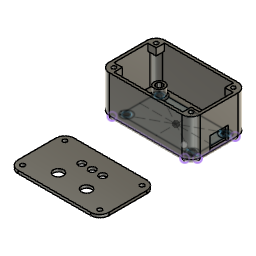
Sound Unit - No Holes (Autodesk Fusion 360 design; units mm, degrees)
Autodesk Fusion 360 part; units mm, degrees
note: some values were not read from the file. Set by a fixed rule: which face or edge a step refers to.
sketch "Sketch1" plane through (0, 0, 0) normal (0, 0, 1) x (1, 0, 0)
  line L0 (6.5, 0) -> (58.5, 0)
  line L1 (65, -6.5) -> (65, -33.5)
  line L2 (58.5, -40) -> (6.5, -40)
  line L3 (0, -33.5) -> (0, -6.5)
  arc A0 (0, -33.5) -> (6.5, -40) centre (6.5, -33.5) ccw
  arc A1 (6.5, 0) -> (0, -6.5) centre (6.5, -6.5) ccw
  arc A2 (65, -6.5) -> (58.5, 0) centre (58.5, -6.5) ccw
  arc A3 (58.5, -40) -> (65, -33.5) centre (58.5, -33.5) ccw
  point P0 (65, 0)
  point P1 (6.5, -33.5)
  point P2 (30.568, -50.8814)
  dimension "d1" = 65
  dimension "d2" = 40
  dimension "d294" = 6.5
  constraint horizontal L0
  constraint vertical L1
  constraint horizontal L2
  constraint vertical L3
  constraint tangent L2 A0
  constraint tangent L3 A0
  constraint coincident origin L0
  constraint coincident origin L3
  constraint tangent L0 A1
  constraint tangent L3 A1
  constraint equal A0 A1
  constraint coincident P0 L0
  constraint coincident P0 L1
  constraint tangent L0 A2
  constraint tangent L1 A2
  constraint equal A0 A2
  constraint tangent L1 A3
  constraint tangent L2 A3
  constraint equal A0 A3
  constraint coincident P1 A0.centre
  measures "d1" distance of origin P0
  measures "d2" distance of L0 L2
  measures "d294" radius of A0
extrude "Extrude1" add sketch "Sketch1" along normal blind 30 makes body 1
sketch "Sketch2" plane through (0, 0, 0) normal (-1, 0, 0) x (0, -1, 0)
shell "Shell1" thickness 2 removed faces 1 at (41.1667, -26.6667, 30) on bodies 1
sketch "Sketch3" plane through (0, 0, 2) normal (0, 0, 1) x (-1, 0, 0)
  circle A0 centre (-10.6, 31.7) radius 2.3971
  line L0 (-60, 6) -> (-60, 34)
  line L1 (-8.3, 34) -> (-8.3, 6)
  circle A1 centre (-57.7, 8.3) radius 3.8971
  circle A2 centre (-10.6, 31.7) radius 3.8971
  line L2 (-60, 34) -> (-8.3, 6) construction
  line L3 (-8.3, 34) -> (-60, 6) construction
  circle A3 centre (-10.6, 8.3) radius 2.3971
  line L4 (-34.15, 6) -> (-34.15, 34) construction
  line L5 (-8.3, 6) -> (-60, 6)
  line L6 (-60, 34) -> (-8.3, 34)
  circle A4 centre (-10.6, 8.3) radius 3.8971
  circle A5 centre (-57.7, 8.3) radius 2.3971
  line L7 (-8.3, 20) -> (-60, 20) construction
  circle A6 centre (-57.7, 31.7) radius 3.8971
  circle A7 centre (-57.7, 31.7) radius 2.3971
  line L8 (-53.8029, 31.6996) -> (-61.5971, 31.6996)
  line L9 (-53.8029, 8.3) -> (-61.5971, 8.3)
  line L10 (-58.5, 38) -> (-6.5, 38)
  line L11 (-63, 6.5) -> (-63, 33.5)
  point P0 (-34.15, 20)
  point P1 (-49.8386, 29.9282)
  dimension "d21" = 51.7
  dimension "d22" = 28
  dimension "d23" = 2.3
  dimension "d24" = 2.3
  dimension "d27" = 1.5
  dimension "d349" = 4
  dimension "d350" = 3
  constraint horizontal L6
  constraint perpendicular L1 L6
  constraint parallel L5 L6
  constraint parallel L0 L1
  constraint coincident P0 L2
  constraint coincident P0 L3
  constraint midpoint L4.start L5
  constraint midpoint L4.end L6
  constraint midpoint L7.start L1
  constraint midpoint L7.end L0
  constraint symmetric A0 A3 L7
  constraint symmetric A3 L4 A5
  constraint symmetric A0 L4 A7
  constraint concentric A3 A4
  constraint symmetric A2 A4 L7
  constraint symmetric A1 L4 A4
  constraint symmetric A2 L4 A6
  constraint coincident A6 L8.start
  constraint coincident A6 L8.end
  constraint perpendicular L0 L8
  constraint coincident A1 L9.start
  constraint coincident A1 L9.end
  constraint horizontal L9
  measures "d21" distance of L1.end L0.start
  measures "d22" distance of L0.start L0.end
  measures "d23" distance of A3.centre L5
  measures "d24" distance of A3.centre L1
  measures "d27" distance of A3 A4
  measures "d349" distance of L6 L10
  measures "d350" distance of L0 L11
extrude "Extrude4" cut sketch "Sketch3" against normal up to surface (2 mm away) contours A0 L1 | A0 L1 L6 | A0 L6 | L1 A3 | L1 A3 L5 | L0 L6 A7 L8 | L6 A7 | A3 L5 | L0 A7 L8 | L0 A7 L8 | L0 A7 L8 | L5 A5 | L0 L5 A5 L9 | L0 A5 L9 | L0 A5 L9 | L0 A5 L9 picked at (-11.2582, 32.2325) picked at (-11.0806, 8.835) bodies 1
extrude "Extrude3" cut sketch "Sketch3" against normal up to surface (1.5 mm away) from surface at -0.5 contours A0 L1 | A0 L1 A2 L6 | A0 L1 L6 | A0 L1 L6 | A0 L1 A2 L6 | A0 L6 | L1 A3 L5 A4 | L1 A3 L5 A4 | L6 A6 A7 L8 | L0 L6 A6 A7 L8 | L1 A3 | L1 A3 L5 | L0 L6 A7 L8 | L6 A7 | L0 A6 A7 L8 | L0 A6 A7 L8 | L1 A3 L5 | A3 L5 | A1 L5 A5 L9 | L0 A1 L5 A5 L9 | L0 L6 A7 | L0 A7 L8 | L0 A7 L8 | L0 A7 L8 | L0 A1 A5 L9 | L0 A1 A5 L9 | L5 A5 | L0 L5 A5 L9 | L0 A5 L9 | L0 A5 L9 | L0 A5 L9 | L0 L5 A5 bodies 1
extrude "Extrude5" add sketch "Sketch3" along normal blind 6.5 contours A0 L1 | A0 L1 A2 L6 | A0 L1 L6 | A0 L1 A2 L6 | A0 L6 | L1 A3 L5 A4 | L1 A3 L5 A4 | L6 A6 A7 L8 | L0 L6 A6 A7 L8 | L1 A3 | L6 A7 | L1 A3 L5 | A3 L5 | A1 L5 A5 L9 | L0 A1 L5 A5 L9 | L0 L6 A7 | L0 A7 L8 | L5 A5 | L0 A5 L9 | L0 L5 A5 picked at (-8.7062, 33.5938) picked at (-8.7062, 6.4062) picked at (-60.0611, 31.7756) picked at (-60.0611, 8.2241) bodies 1
chamfer "Chamfer1" distance 1 angle 45 4 edges at (14.2334, -9.7092, 2) (14.2334, -33.1092, 2) (57.7, -35.5971, 2) (57.7, -4.4029, 2) on bodies 1
sketch "Sketch5" plane through (63, 0, 0) normal (-1, 0, 0) x (0, -1, 0)
  line L0 (33.5, 30) -> (6.5, 30)
  line L1 (13.5, 13.5, -2) -> (26.5, 13.5, -2)
  line L2 (26.5, 13.5, -2) -> (26.5, 3.5, -2)
  line L3 (26.5, 3.5, -2) -> (13.5, 3.5, -2)
  line L4 (13.5, 3.5, -2) -> (13.5, 13.5, -2)
  line L5 (26.5, 13.5, -2) -> (13.5, 3.5, -2) construction
  line L6 (26.5, 3.5, -2) -> (13.5, 13.5, -2) construction
  line L7 (33.5, 0) -> (33.5, 30)
  line L8 (33.5, 30, -2) -> (6.5, 0, -2) construction
  line L9 (6.5, 0, -2) -> (6.5, 30, -2) construction
  line L10 (6.5, 30, -2) -> (33.5, 0, -2) construction
  line L11 (6.5, 2) -> (33.5, 2)
  line L12 (6.5, 0, -2) -> (33.5, 0, -2)
  point P0 (20, 12.5)
  point P1 (33.5, 30)
  point P2 (6.5, 0)
  point P3 (6.5, 30)
  point P4 (33.5, 0)
  point P5 (20, 12.5)
  dimension "d46" = 13
  dimension "d47" = 10
  dimension "d356" = 3.5
  constraint coincident P1 L0.start
  constraint coincident P3 L0.end
  constraint coincident P4 L7.start
  constraint coincident P5 P0
extrude "Extrude13" cut sketch "Sketch5" along normal up to surface (2 mm away) contours L1 L2 L3 L4 in plane through (65, 0, 0) normal (-1, 0, 0) bodies 1
sketch "Sketch6" plane through (0, -40, 0) normal (0, -1, 0) x (1, 0, 0)
  line L0 (58.5, 30) -> (6.5, 30)
  line L1 (60, 2) -> (8.3, 2)
  line L2 (6.5, 0) -> (58.5, 0)
  line L3 (58.5, 0) -> (58.5, 30)
  line L4 (6.5, 30) -> (6.5, 0)
sketch "Sketch7" plane through (0, 0, 30) normal (0, 0, 1) x (-1, 0, 0)
  arc A0 (-6.5, 0) -> (0, 6.5) centre (-6.5, 6.5) ccw construction
  circle A1 centre (-4.9038, 4.9038) radius 1.5
  arc A2 (-6.5, 2) -> (-2, 6.5) centre (-6.5, 6.5) ccw
  line L0 (-1.9038, 1.9038) -> (-7.9038, 1.9038) construction
  line L1 (-7.9038, 1.9038) -> (-7.9038, 7.9038) construction
  line L2 (-7.9038, 7.9038) -> (-1.9038, 7.9038) construction
  line L3 (-1.9038, 7.9038) -> (-1.9038, 1.9038) construction
  line L4 (-1.9038, 1.9038) -> (-7.9038, 7.9038) construction
  line L5 (-1.9038, 7.9038) -> (-7.9038, 1.9038) construction
  line L6 (-7.9038, 7.9038) -> (-2, 7.9038)
  line L7 (-7.9038, 2) -> (-7.9038, 7.9038)
  line L8 (-7.9038, 2) -> (-6.5, 2)
  line L9 (-2, 7.9038) -> (-2, 6.5)
  line L10 (-63.0962, 1.9038) -> (-57.0962, 1.9038) construction
  line L11 (-57.0962, 1.9038) -> (-57.0962, 7.9038) construction
  line L12 (-57.0962, 7.9038) -> (-63.0962, 7.9038) construction
  line L13 (-63.0962, 7.9038) -> (-63.0962, 1.9038) construction
  arc A3 (-65, 6.5) -> (-58.5, 0) centre (-58.5, 6.5) ccw construction
  line L14 (-57.0962, 7.9038) -> (-63.0962, 1.9038) construction
  line L15 (-57.0962, 1.9038) -> (-63.0962, 7.9038) construction
  circle A4 centre (-60.0962, 4.9038) radius 1.5
  line L16 (-57.0962, 2) -> (-57.0962, 7.9038)
  line L17 (-63, 7.9038) -> (-57.0962, 7.9038)
  line L18 (-63, 7.9038) -> (-63, 6.5)
  line L19 (-57.0962, 2) -> (-58.5, 2)
  arc A5 (-63, 6.5) -> (-58.5, 2) centre (-58.5, 6.5) ccw
  line L20 (-63.0962, 38.0962) -> (-57.0962, 38.0962) construction
  line L21 (-57.0962, 38.0962) -> (-57.0962, 32.0962) construction
  line L22 (-57.0962, 32.0962) -> (-63.0962, 32.0962) construction
  line L23 (-63.0962, 32.0962) -> (-63.0962, 38.0962) construction
  arc A6 (-58.5, 40) -> (-65, 33.5) centre (-58.5, 33.5) ccw construction
  line L24 (-63.0962, 32.0962) -> (-57.0962, 38.0962) construction
  line L25 (-57.0962, 32.0962) -> (-63.0962, 38.0962) construction
  circle A7 centre (-60.0962, 35.0962) radius 1.5
  line L26 (-57.0962, 32.0962) -> (-63.0227, 32.0962)
  line L27 (-63.0227, 32.0962) -> (-63, 33.5)
  line L28 (-57.0962, 32.0962) -> (-57.0962, 38.007)
  line L29 (-57.0962, 38.007) -> (-58.5, 38)
  arc A8 (-58.5, 38) -> (-63, 33.5) centre (-58.5, 33.5) ccw
  line L30 (-1.9038, 38.0962) -> (-7.9038, 38.0962) construction
  line L31 (-7.9038, 38.0962) -> (-7.9038, 32.0962) construction
  line L32 (-7.9038, 32.0962) -> (-1.9038, 32.0962) construction
  line L33 (-1.9038, 32.0962) -> (-1.9038, 38.0962) construction
  arc A9 (0, 33.5) -> (-6.5, 40) centre (-6.5, 33.5) ccw construction
  line L34 (-1.9038, 38.0962) -> (-7.9038, 32.0962) construction
  line L35 (-1.9038, 32.0962) -> (-7.9038, 38.0962) construction
  circle A10 centre (-4.9038, 35.0962) radius 1.5
  line L36 (-7.9038, 32.0962) -> (-2, 32.0962)
  line L37 (-2, 32.0962) -> (-2, 33.5)
  line L38 (-7.9038, 32.0962) -> (-7.9038, 38.1423)
  line L39 (-7.9038, 38.1423) -> (-6.5, 38)
  arc A11 (-2, 33.5) -> (-6.5, 38) centre (-6.5, 33.5) ccw
  point P0 (-9.5, -1)
  point P1 (-3.318, 3.318)
  point P2 (-4.9038, 4.9038)
  point P3 (-4.9038, 4.9038)
  point P4 (-3.318, 3.318)
  point P5 (-3.724, 2.9583)
  point P6 (-60.0962, 4.9038)
  point P7 (-58.5, 2)
  point P8 (-63, 6.5)
  point P9 (-61.682, 3.318)
  point P10 (-77.5, 3.8)
  point P11 (-60.0962, 35.0962)
  point P12 (-63, 33.5)
  point P13 (-58.5, 38)
  point P14 (-61.682, 36.682)
  point P15 (-4.9038, 35.0962)
  point P16 (-2, 33.5)
  point P17 (-6.5, 38)
  point P18 (-3.318, 36.682)
  point P19 (-2, 53.1422)
  dimension "d309" = 3
  dimension "d322" = 6
  dimension "d323" = 6
  dimension "d324" = 6
  dimension "d325" = 6
  dimension "d326" = 3
  dimension "d329" = 6
  dimension "d330" = 6
  dimension "d331" = 3
  dimension "d332" = 6
  dimension "d333" = 6
  dimension "d334" = 3
  constraint midpoint P4 A2
  constraint coincident P3 P2
  constraint horizontal L0
  constraint vertical L1
  constraint horizontal L2
  constraint vertical L3
  constraint midpoint A0 L0.start
  constraint midpoint L5 P3
  constraint coincident L2 L6.end
  constraint coincident L1 L7.start
  constraint coincident P4 P1
  constraint coincident A2.start L8.end
  constraint tangent A2 L8
  constraint coincident A2.end L9.end
  constraint tangent A2 L9
  constraint horizontal L10
  constraint vertical L11
  constraint horizontal L12
  constraint vertical L13
  constraint midpoint L10.start A3
  constraint midpoint L15 P6
  constraint coincident P6 A4.centre
  constraint coincident L11 L16.start
  constraint coincident L12 L17.start
  constraint perpendicular L16 L17
  constraint coincident P8 L18.end
  constraint perpendicular L17 L18
  constraint coincident P7 L19.end
  constraint perpendicular L16 L19
  constraint midpoint P9 A5
  constraint horizontal L20
  constraint vertical L21
  constraint horizontal L22
  constraint vertical L23
  constraint midpoint L20.start A6
  constraint midpoint L24 P11
  constraint coincident P11 A7.centre
  constraint coincident L22 L26.end
  constraint coincident P12 L27.end
  constraint coincident L21 L28.end
  constraint coincident P13 L29.end
  constraint midpoint P14 A8
  constraint horizontal L30
  constraint vertical L31
  constraint horizontal L32
  constraint vertical L33
  constraint midpoint L30.start A9
  constraint midpoint L34 P15
  constraint coincident P15 A10.centre
  constraint coincident L32 L36.end
  constraint coincident P16 L37.end
  constraint coincident L31 L38.end
  constraint perpendicular L32 L38
  constraint coincident P17 L39.end
  constraint midpoint P18 A11
  measures "d309" diameter of A1
  measures "d322" distance of L0.start L0.end
  measures "d323" distance of L0.start L2.end
  measures "d324" distance of L10.start L10.end
  measures "d325" distance of L10.start L12.end
  measures "d326" diameter of A4
  measures "d329" distance of L20.start L20.end
  measures "d330" distance of L20.start L22.end
  measures "d331" diameter of A7
  measures "d332" distance of L30.start L30.end
  measures "d333" distance of L30.start L32.end
  measures "d334" diameter of A10
extrude "Extrude8" add sketch "Sketch7" against normal blind 5 bodies 1
sketch "Sketch8" plane through (0, 0, 0) normal (0, 0, 1) x (1, 0, 0)
  line L0 (58.3615, -65.1296) -> (6.3615, -65.1296)
  line L1 (-0.1385, -71.6296) -> (-0.1385, -98.6296)
  line L2 (6.3615, -105.1296) -> (58.3615, -105.1296)
  line L3 (64.8615, -98.6296) -> (64.8615, -71.6296)
  arc A0 (6.3615, -65.1296) -> (-0.1385, -71.6296) centre (6.3615, -71.6296) ccw
  arc A1 (-0.1385, -98.6296) -> (6.3615, -105.1296) centre (6.3615, -98.6296) ccw
  arc A2 (64.8615, -71.6296) -> (58.3615, -65.1296) centre (58.3615, -71.6296) ccw
  arc A3 (58.3615, -105.1296) -> (64.8615, -98.6296) centre (58.3615, -98.6296) ccw
  line L4 (1.7653, -67.0334) -> (62.9576, -103.2258) construction
  line L5 (62.9576, -67.0334) -> (1.7653, -103.2258) construction
  circle A4 centre (4.7653, -70.0334) radius 1.5
  line L6 (1.7653, -67.0334) -> (7.7653, -67.0334) construction
  line L7 (7.7653, -67.0334) -> (7.7653, -73.0334) construction
  line L8 (7.7653, -73.0334) -> (1.7653, -73.0334) construction
  line L9 (1.7653, -73.0334) -> (1.7653, -67.0334) construction
  line L10 (7.7653, -67.0334) -> (1.7653, -73.0334) construction
  line L11 (1.7653, -67.0334) -> (7.7653, -73.0334) construction
  line L12 (62.9576, -67.0334) -> (56.9576, -67.0334) construction
  line L13 (56.9576, -67.0334) -> (56.9576, -73.0334) construction
  line L14 (56.9576, -73.0334) -> (62.9576, -73.0334) construction
  line L15 (62.9576, -73.0334) -> (62.9576, -67.0334) construction
  line L16 (56.9576, -67.0334) -> (62.9576, -73.0334) construction
  line L17 (56.9576, -73.0334) -> (62.9576, -67.0334) construction
  circle A5 centre (59.9576, -70.0334) radius 1.5
  line L18 (62.9576, -103.2258) -> (56.9576, -103.2258) construction
  line L19 (56.9576, -103.2258) -> (56.9576, -97.2258) construction
  line L20 (56.9576, -97.2258) -> (62.9576, -97.2258) construction
  line L21 (62.9576, -97.2258) -> (62.9576, -103.2258) construction
  line L22 (56.9576, -97.2258) -> (62.9576, -103.2258) construction
  line L23 (62.9576, -97.2258) -> (56.9576, -103.2258) construction
  circle A6 centre (59.9576, -100.2258) radius 1.5
  line L24 (1.7653, -103.2258) -> (7.7653, -103.2258) construction
  line L25 (7.7653, -103.2258) -> (7.7653, -97.2258) construction
  line L26 (7.7653, -97.2258) -> (1.7653, -97.2258) construction
  line L27 (1.7653, -97.2258) -> (1.7653, -103.2258) construction
  line L28 (1.7653, -97.2258) -> (7.7653, -103.2258) construction
  line L29 (7.7653, -97.2258) -> (1.7653, -103.2258) construction
  circle A7 centre (4.7653, -100.2258) radius 1.5
  line L30 (20.1684, -78.0671) -> (44.5545, -78.0671) construction
  circle A8 centre (22.2882, -92.1922) radius 3.65
  circle A9 centre (24.8615, -78.0671) radius 2.5
  circle A10 centre (32.3615, -78.0671) radius 2.5
  circle A11 centre (39.8615, -78.0671) radius 2.5
  circle A12 centre (42.4347, -92.1922) radius 3.65
  line L31 (-0.1385, -85.1296) -> (64.8615, -85.1296) construction
  line L32 (32.3615, -65.1296) -> (32.3615, -105.1296) construction
  line L33 (22.2882, -92.1922) -> (42.4347, -92.1922) construction
  line L34 (32.3615, -78.0671) -> (32.3615, -92.1922) construction
  point P0 (4.7653, -70.0334)
  point P1 (59.9576, -70.0334)
  point P2 (59.9576, -100.2258)
  point P3 (4.7653, -100.2258)
  point P4 (32.3615, -85.1296)
  dimension "d179" = 6.5
  dimension "d196" = 40
  dimension "d197" = 65
  dimension "d303" = 3
  dimension "d336" = 6
  dimension "d337" = 6
  dimension "d338" = 6
  dimension "d339" = 6
  dimension "d340" = 3
  dimension "d341" = 6
  dimension "d342" = 6
  dimension "d343" = 3
  dimension "d344" = 6
  dimension "d345" = 6
  dimension "d346" = 3
  dimension "d370" = 5
  dimension "d371" = 5
  dimension "d372" = 5
  dimension "d373" = 7.5
  dimension "d374" = 7.5
  constraint horizontal L0
  constraint vertical L1
  constraint horizontal L2
  constraint vertical L3
  constraint tangent L0 A0
  constraint tangent L1 A0
  constraint tangent L1 A1
  constraint tangent L2 A1
  constraint equal A0 A1
  constraint tangent L0 A2
  constraint tangent L3 A2
  constraint equal A0 A2
  constraint tangent L2 A3
  constraint tangent L3 A3
  constraint equal A0 A3
  constraint midpoint A1 L5.end
  constraint midpoint A0 L4.start
  constraint midpoint A2 L5.start
  constraint midpoint A3 L4.end
  constraint horizontal L6
  constraint vertical L7
  constraint horizontal L8
  constraint vertical L9
  constraint midpoint L10 P0
  constraint coincident P0 A4.centre
  constraint horizontal L12
  constraint vertical L13
  constraint horizontal L14
  constraint vertical L15
  constraint midpoint L17 P1
  constraint coincident P1 A5.centre
  constraint horizontal L18
  constraint vertical L19
  constraint horizontal L20
  constraint vertical L21
  constraint midpoint L22 P2
  constraint coincident P2 A6.centre
  constraint horizontal L24
  constraint vertical L25
  constraint horizontal L26
  constraint vertical L27
  constraint midpoint L28 P3
  constraint coincident P3 A7.centre
  constraint midpoint L5 P4
  constraint midpoint A10.centre L30
  constraint coincident A9.centre L30
  constraint coincident A11.centre L30
  constraint midpoint L1 L31.start
  constraint midpoint L3 L31.end
  constraint midpoint L0 L32.start
  constraint midpoint L2 L32.end
  constraint coincident A8.centre L33.start
  constraint coincident A12.centre L33.end
  constraint parallel L30 L33
  constraint coincident A10.centre L34.start
  constraint midpoint L33 L34.end
  constraint perpendicular L33 L34
  constraint parallel L32 L34
  constraint midpoint P4 L34
  measures "d179" radius of A0
  measures "d196" distance of L0 L2
  measures "d197" distance of L1 L3
  measures "d303" diameter of A4
  measures "d336" distance of L4.start L6.end
  measures "d337" distance of L4.start L8.end
  measures "d338" distance of L5.start L12.end
  measures "d339" distance of L5.start L14.end
  measures "d340" diameter of A5
  measures "d341" distance of L4.end L18.end
  measures "d342" distance of L4.end L20.end
  measures "d343" diameter of A6
  measures "d344" distance of L5.end L24.end
  measures "d345" distance of L5.end L26.end
  measures "d346" diameter of A7
  measures "d370" diameter of A10
  measures "d371" diameter of A9
  measures "d372" diameter of A11
  measures "d373" distance of A10.centre A11.centre
  measures "d374" distance of A10.centre A9.centre
extrude "Extrude10" add sketch "Sketch8" along normal blind 2 separate body contours L0 L1 L2 L3 A0 A1 A2 A3 | A8 | A9 | A10 | A11 | A12 makes body 2
sketch "Sketch10" plane through (0, 0, 0) normal (0, 1, 0) x (-1, 0, 0)
  line L0 (-6.5, 30) -> (-58.5, 30)
  line L1 (-58.5, 30) -> (8.3532, 2.6385) construction
  line L2 (-6.5, 30) -> (-73.5, 3) construction
  line L3 (-73.4991, 16.2746) -> (-40.0734, 16.3193) construction
  line L4 (-40.0734, 16.3193) -> (-6.574, 16.5124) construction
  line L5 (-58.5, 0) -> (-6.5, 0)
  line L6 (-6.5, 0) -> (-6.5, 30)
  line L7 (-58.5, 30) -> (-58.5, 0)
  dimension "d283" = 72.2357
  dimension "d284" = 72.2357
  dimension "d286" = 33.5
  constraint coincident L0.end L1.start
  constraint coincident L0.start L2.start
  measures "d283" distance of L0.end L1.end
  measures "d284" distance of L0.start L2.end
  measures "d286" distance of L3.end L4.end
fillet "Fillet3" radius 3.5 8 edges at (1.9038, -1.9038, 0) (32.5, 0, 0) (63.0962, -1.9038, 0) (65, -20, 0) (63.0962, -38.0962, 0) (32.5, -40, 0) (1.9038, -38.0962, 0) (0, -20, 0) on bodies 1
sketch "Sketch11" plane through (0, 0, 0) normal (0, 1, 0) x (-1, 0, 0)
  line L0 (-58.5, 3.5) -> (-6.5, 3.5)
  line L1 (-6.5, 3.5) -> (-6.5, 30)
  line L2 (-6.5, 30) -> (-58.5, 30)
  line L3 (-58.5, 30) -> (-58.5, 3.5)
extrude "Extrude15" cut sketch "Sketch8" along normal blind 2 contours A8 | A9 | A10 | A11 | A12 bodies 2
equation "d23 = 0.8 mm + 1.5 mm"
equation "d116 = 6.5 mm + 3.5 mm"
named bodies: "Casing"
